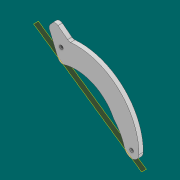
# Autodesk Inventor part: canere_02_t3_01
Saved by Autodesk Inventor 2022 (Build 260153000, 153)
## iProperties
Created: 2023-06-03
Part Number: canere_02_t3_01
Material: 一般
Document SubType Name: Modeling
Designer: nyxeon
Density: 1 g/cm^3
Appearance: 既定
Author: nyxeon
Autodesk Inventor part; units mm, degrees
ref_plane "YZ Plane" through (0, 0, 0) normal (1, 0, 0) x (0, 1, 0)
ref_plane "XZ Plane" through (0, 0, 0) normal (0, 1, 0) x (-1, 0, 0)
ref_plane "XY Plane" through (0, 0, 0) normal (0, 0, 1) x (1, 0, 0)
sketch "スケッチ1" plane through (0, 0, 0) normal (0, 0, 1) x (1, 0, 0)
  circle A0 centre (0, 0) radius 33.5 construction
  circle A1 centre (0, 0) radius 43.5
  dimension "d0" = 67
  dimension "d1" = 87
  constraints: 2 centre point, 2 coincident
  measures "d0" diameter of A0
  measures "d1" diameter of A1
extrude "押し出し1" add sketch "スケッチ1" along normal blind 1
sketch "スケッチ2" plane through (0, 0, 1) normal (0, 0, 1) x (1, 0, 0)
  circle A0 centre (0, 0) radius 33.5
  circle A1 centre (0, 0) radius 43.5 projected
  dimension "d4" = 67
  constraints: 1 centre point, 1 coincident
  measures "d4" diameter of A0
extrude "押し出し2" add sketch "スケッチ2" along normal blind 2
sketch "スケッチ4" plane through (0, 0, 3) normal (0, 0, 1) x (1, 0, 0)
  circle A0 centre (0, 0) radius 33.5 construction
  circle A1 centre (0, 0) radius 43.5 construction
  line L0 (0, 0) -> (33.5, 0) construction
  line L1 (33.5, 0) -> (43.5, 0) construction
  circle A2 centre (0, 0) radius 33.5 construction
  line L2 (0, 0) -> (-33.5, 0) construction
  circle A3 centre (0, 0) radius 43.5 construction
  line L3 (-43.5, 0) -> (-33.5, 0) construction
  circle A4 centre (38.5, 0) radius 3.05
  circle A5 centre (-38.5, 0) radius 3.05
  circle A6 centre (0, 0) radius 38.5 construction
  circle A7 centre (-9.9645, 37.1881) radius 3.05 construction
  arc A8 (-3.4944, 44.3648) -> (-9.9645, 37.1881) centre (38.5, 0) ccw construction
  line L4 (38.5, 0) -> (-9.9645, 37.1881) construction
  line L5 (-9.9645, 37.1881) -> (-12.3843, 39.0449) construction
  arc A9 (0.0788, 43.4999) -> (-7.5448, 35.3314) centre (38.5, 0) ccw
  arc A10 (-9.6001, 42.4274) -> (-12.3843, 39.0449) centre (38.5, 0) ccw
  arc A11 (-12.3843, 39.0449) -> (-7.5448, 35.3314) centre (-9.9645, 37.1881) ccw
  arc A12 (0.0788, 43.4999) -> (-9.6001, 42.4274) centre (0, 0) ccw
  circle A13 centre (9.9645, -37.1881) radius 3.05 construction
  line L6 (-38.5, 0) -> (9.9645, -37.1881) construction
  line L7 (9.9645, -37.1881) -> (12.3843, -39.0449) construction
  arc A14 (-0.0788, -43.4999) -> (7.5448, -35.3314) centre (-38.5, 0) ccw
  arc A15 (9.6001, -42.4274) -> (12.3843, -39.0449) centre (-38.5, 0) ccw
  arc A16 (12.3843, -39.0449) -> (7.5448, -35.3314) centre (9.9645, -37.1881) ccw
  arc A17 (-0.0788, -43.4999) -> (9.6001, -42.4274) centre (0, 0) ccw
  line L8 (-9.9645, 37.1881) -> (9.9645, -37.1881) construction
  dimension "d7" = 6.1
  dimension "d8" = 3.05
  dimension "d15" = 105
  constraints: 31 point on circle, 18 end point, 14 centre point, 11 coincident, 7 point on line, 3 midpoint, 2 equal radius, 1 collinear, 1 horizontal, 1 horizontal alignment, 1 other
  measures "d7" diameter of A4
  measures "d8" radius of A11
  measures "d15" angle of L0 L8
extrude "押し出し3" cut sketch "スケッチ4" against normal through all
fillet "フィレット1" radius 1 4 edges at (-9.6001, 42.4274, 1.5) (0.0788, 43.4999, 1.5) (-0.0788, -43.4999, 1.5) (9.6001, -42.4274, 1.5)
sketch "スケッチ6" plane through (0, 0, 3) normal (0, 0, 1) x (1, 0, 0)
  arc A0 (-12.3843, 39.0449) -> (-7.5448, 35.3314) centre (-9.9645, 37.1881) ccw construction
  circle A1 centre (38.5, 0) radius 3.05 construction
  circle A2 centre (-9.9645, 37.1881) radius 3
  circle A3 centre (38.5, 0) radius 3
  point P0 (0, 0)
  dimension "d16" = 6
  constraints: 2 centre point, 2 coincident, 1 equal radius
  measures "d16" diameter of A2
extrude "押し出し5" add sketch "スケッチ6" along normal blind 0.1
sketch "スケッチ7" plane through (-9.9645, 37.1881, 3.1) normal (0, 0, 1) x (1, 0, 0)
  circle A0 centre (0, 0) radius 3 construction
  circle A1 centre (48.4645, -37.1881) radius 3 construction
  circle A2 centre (0, 0) radius 5
  circle A3 centre (48.4645, -37.1881) radius 3 projected
  circle A4 centre (48.4645, -37.1881) radius 5
  point P0 (9.9645, -37.1881)
  dimension "d19" = 10
  constraints: 2 centre point, 2 coincident, 1 equal radius
  measures "d19" diameter of A2
extrude "押し出し6" add sketch "スケッチ7" along normal blind 0.4 contours A2 | A3 | A4
sketch "スケッチ8" plane through (-9.9645, 37.1881, 3.5) normal (0, 0, 1) x (1, 0, 0)
  circle A0 centre (9.9645, -37.1881) radius 33.5 construction
  circle A1 centre (9.9645, -37.1881) radius 29 construction
  circle A2 centre (48.4645, -37.1881) radius 5 construction
  arc A3 (43.6349, -38.4822) -> (36.1372, -24.6985) centre (11.2764, -47.1527) ccw construction
  line L0 (9.9645, -37.1881) -> (48.4645, -37.1881) construction
  line L1 (48.4645, -37.1881) -> (11.2764, -47.1527) construction
  circle A4 centre (0, 0) radius 5 construction
  circle A5 centre (48.4645, -37.1881) radius 3.05 construction
  line L2 (48.4645, -37.1881) -> (-9.5202, 7.3051) construction
  line L3 (9.9645, -37.1881) -> (-4.6207, -1.9104) construction
  circle A6 centre (0, 0) radius 5 construction
  line L4 (-1.1156, -10.3883) -> (-7.9245, 6.0806)
  arc A7 (36.1372, -24.6985) -> (-1.1156, -10.3883) centre (9.9645, -37.1881) ccw
  arc A8 (43.6349, -38.4822) -> (36.1372, -24.6985) centre (11.2764, -47.1527) ccw
  arc A9 (22.6521, -78.7967) -> (10.4317, 6.3093) centre (9.9645, -37.1881) ccw projected
  arc A10 (43.6349, -38.4822) -> (53.4645, -37.1881) centre (48.4645, -37.1881) ccw
  arc A11 (53.4645, -37.1881) -> (5.2496, 6.0556) centre (9.9645, -37.1881) ccw
  line L5 (-7.9245, 6.0806) -> (-9.5202, 7.3051)
  line L6 (-9.5202, 7.3051) -> (-4.6501, 13.652)
  line L7 (-4.6501, 13.652) -> (5.2496, 6.0556)
  point P0 (10.4317, 6.3093)
  dimension "d22" = 58
  dimension "d23" = 15
  dimension "d24" = 12
  dimension "d25" = 8
  constraints: 18 point on circle, 16 end point, 6 centre point, 5 coincident, 5 point on line, 2 perpendicular, 2 tangent, 1 collinear, 1 equal radius, 1 horizontal, 2 other
  measures "d22" diameter of A1
  measures "d23" angle of L1 L0
  measures "d24" distance of A4.centre L2.end
  measures "d25" distance of L2.end L6.end
extrude "押し出し7" add sketch "スケッチ8" along normal blind 2.5
sketch "スケッチ9" plane through (0, 0, 3) normal (0, 0, 1) x (1, 0, 0)
  circle A0 centre (0, 0) radius 61.8319
  constraints: 1 centre point, 1 coincident
extrude "押し出し8" cut sketch "スケッチ9" against normal through all
sketch "スケッチ10" plane through (-9.9645, 37.1881, 3) normal (0, 0, -1) x (-1, 0, 0)
  circle A0 centre (-48.4645, -37.1881) radius 3 construction
  circle A1 centre (0, 0) radius 3 construction
  circle A2 centre (-48.4645, -37.1881) radius 1.3
  circle A3 centre (0, 0) radius 1.3
  point P0 (-9.9645, -37.1881)
  dimension "d30" = 2.6
  constraints: 2 centre point, 2 coincident, 1 equal radius
  measures "d30" diameter of A2
extrude "押し出し9" cut sketch "スケッチ10" against normal through all
fillet "フィレット2" radius 3 6 edges at (-19.4848, 44.4933, 4.75) (-14.6147, 50.8401, 4.75) (-17.889, 43.2688, 4.75) (-4.7149, 43.2437, 4.75) (-11.0801, 26.7998, 4.75) (26.1727, 12.4896, 4.75)
sketch "スケッチ11" plane through (38.5, 0, 3) normal (0, 0, -1) x (-1, 0, 0)
  circle A0 centre (0, 0) radius 3 projected
  circle A1 centre (0, 0) radius 5 projected
  circle A2 centre (48.4645, 37.1881) radius 3 projected
  circle A3 centre (48.4645, 37.1881) radius 5 projected
  point P0 (38.5, 0)
extrude "押し出し10" add sketch "スケッチ11" against normal up to surface (0.1 mm away)
sketch "スケッチ12" plane through (-9.9645, 37.1881, 3.5) normal (0, 0, -1) x (-1, 0, 0)
  arc A0 (7.9351, 5.9159) -> (7.8609, 9.4676) centre (5.4809, 7.6413) ccw projected
  line L0 (6.4764, 11.2719) -> (7.8609, 9.4676) projected
  arc A1 (6.4764, 11.2719) -> (2.2701, 11.8257) centre (4.0964, 9.4456) ccw projected
  line L1 (-4.3131, 6.7742) -> (2.2701, 11.8257) projected
  arc A2 (-6.3862, 6.1644) -> (-4.3131, 6.7742) centre (-6.1394, 9.1543) ccw projected
  arc A3 (-6.3862, 6.1644) -> (-53.4645, -37.1881) centre (-9.9645, -37.1881) ccw projected
  arc A4 (-43.6349, -38.4822) -> (-53.4645, -37.1881) centre (-48.4645, -37.1881) ccw projected
  arc A5 (-36.4032, -24.9966) -> (-43.6349, -38.4822) centre (-11.2764, -47.1527) ccw projected
  arc A6 (-36.4032, -24.9966) -> (-35.9638, -24.3414) centre (-38.6534, -23.0124) ccw projected
  arc A7 (-1.4457, -9.4676) -> (-35.9638, -24.3414) centre (-9.9645, -37.1881) ccw projected
  arc A8 (-1.4457, -9.4676) -> (2.2079, -7.7461) centre (-0.5645, -6.5999) ccw projected
  line L2 (4.6207, -1.9104) -> (2.2079, -7.7461) projected
  circle A9 centre (0, 0) radius 5 projected
  line L3 (7.6169, 5.3368) -> (4.6207, -1.9104) projected
  arc A10 (7.9351, 5.9159) -> (7.6169, 5.3368) centre (10.3893, 4.1906) ccw projected
  constraints: 1 other
extrude "押し出し11" add sketch "スケッチ12" along normal up to surface (0.5 mm away)
ref_plane "作業平面1" through (-8.5188, 27.7206, 3.5) normal (-0.5666562, -0.8239543, 0) x (0, 0, -1)
